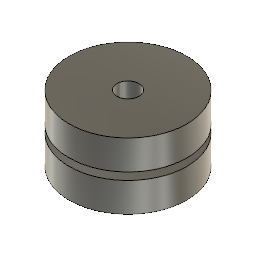
Drive_Wheel (Autodesk Fusion 360 design; units mm, degrees)
Autodesk Fusion 360 part; units mm, degrees
sketch "Sketch1" plane through (0, 0, 0) normal (0, 0, 1) x (1, 0, 0)
  circle A0 centre (0, 0) radius 2
  dimension "d1" = 4
  constraint coincident A0.centre origin
  measures "d1" diameter of A0
extrude "Extrude1" add sketch "Sketch1" along normal blind 1 makes body 1
sketch "Sketch2" plane through (0, 0, 1) normal (0, 0, 1) x (-1, 0, 0)
  circle A0 centre (0, 0) radius 2
  circle A1 centre (0, 0) radius 1.375
  dimension "d4" = 2.75
  constraint coincident A0.centre A1.centre
  measures "d4" diameter of A1
extrude "Extrude2" add sketch "Sketch2" along normal blind 0.25 contours A1 bodies 1
sketch "Sketch3" plane through (0, 0, 0) normal (0, 0, 1) x (1, 0, 0)
  circle A0 centre (0, 0) radius 1.5
  circle A1 centre (0, 0) radius 2
  dimension "d7" = 3
  dimension "d8" = 4
  constraint coincident A0.centre A1.centre
  measures "d7" diameter of A0
  measures "d8" diameter of A1
extrude "Extrude3" add sketch "Sketch3" along normal blind 2.25 and the other way blind -1.25 separate body contours A0 | A1 makes body 2
hole "Hole1" at (0, 0, 2.25) direction (0, 0, -1) diameter 0.75 depth 2.1 tip angle 118 bodies 1 2
